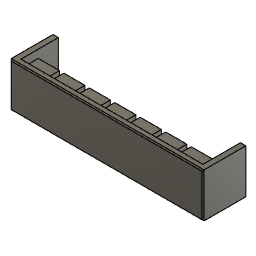
Mornsun PSU Cover (Autodesk Fusion 360 design; units mm, degrees)
Autodesk Fusion 360 part; units mm, degrees
sketch "Sketch1" plane through (0, 0, 0) normal (0, 0, 1) x (1, 0, 0) in component "Cover"
  line L0 (34, 8.25) -> (-34, 8.25)
  line L1 (-34, 8.25) -> (-34, -8.25)
  line L2 (-34, -8.25) -> (34, -8.25)
  line L3 (34, -8.25) -> (34, 8.25)
  line L4 (34, 8.25) -> (-34, -8.25) construction
  line L5 (-34, 8.25) -> (34, -8.25) construction
  line L6 (-32.5, -6.75) -> (32.5, -6.75) construction
  line L7 (32.5, -6.75) -> (32.5, 6.75) construction
  line L8 (32.5, 6.75) -> (-32.5, 6.75)
  line L9 (-32.5, 6.75) -> (-32.5, -6.75) construction
  line L10 (32.5, 4.25) -> (24.6, 4.25)
  line L11 (24.6, 4.25) -> (24.6, 6.75)
  line L12 (24.6, 6.75) -> (32.5, 6.75)
  line L13 (32.5, 6.75) -> (32.5, 4.25)
  line L14 (22.9833, 6.75) -> (22.9833, 4.25)
  line L15 (15.0833, 4.25) -> (15.0833, 6.75)
  line L16 (22.9833, 4.25) -> (15.0833, 4.25)
  line L17 (15.0833, 6.75) -> (22.9833, 6.75)
  line L18 (13.4667, 6.75) -> (13.4667, 4.25)
  line L19 (5.5667, 4.25) -> (5.5667, 6.75)
  line L20 (13.4667, 4.25) -> (5.5667, 4.25)
  line L21 (5.5667, 6.75) -> (13.4667, 6.75)
  line L22 (3.95, 6.75) -> (3.95, 4.25)
  line L23 (-3.95, 4.25) -> (-3.95, 6.75)
  line L24 (3.95, 4.25) -> (-3.95, 4.25)
  line L25 (-3.95, 6.75) -> (3.95, 6.75)
  line L26 (-5.5667, 6.75) -> (-5.5667, 4.25)
  line L27 (-13.4667, 4.25) -> (-13.4667, 6.75)
  line L28 (-5.5667, 4.25) -> (-13.4667, 4.25)
  line L29 (-13.4667, 6.75) -> (-5.5667, 6.75)
  line L30 (-15.0833, 6.75) -> (-15.0833, 4.25)
  line L31 (-22.9833, 4.25) -> (-22.9833, 6.75)
  line L32 (-15.0833, 4.25) -> (-22.9833, 4.25)
  line L33 (-22.9833, 6.75) -> (-15.0833, 6.75)
  line L34 (-24.6, 6.75) -> (-24.6, 4.25)
  line L35 (-32.5, 4.25) -> (-32.5, 6.75)
  line L36 (-24.6, 4.25) -> (-32.5, 4.25)
  line L37 (-32.5, 6.75) -> (-24.6, 6.75)
  line L38 (-34, -8.25) -> (-36, -8.25)
  line L39 (-36, -8.25) -> (-36, 8.25)
  line L40 (-36, 8.25) -> (-34, 8.25)
  line L41 (-34, 8.25) -> (-34, -8.25)
  line L42 (34, -8.25) -> (36, -8.25)
  line L43 (36, -8.25) -> (36, 8.25)
  line L44 (36, 8.25) -> (34, 8.25)
  line L45 (34, 8.25) -> (34, -8.25)
  dimension "d39" = 68
  dimension "d40" = 16.5
  dimension "d42" = 7.9
  dimension "d43" = 2.5
  dimension "d46" = -57.1
  dimension "d47" = 0
  dimension "d52" = 2
  dimension "d53" = 2
  constraint horizontal L0
  constraint perpendicular L0 L1
  constraint parallel L0 L2
  constraint parallel L1 L3
  constraint coincident L4 origin
  constraint coincident L5 origin
  constraint horizontal L10
  constraint vertical L11
  constraint horizontal L12
  constraint vertical L13
  constraint coincident L8 L11.end
  constraint coincident L7 L10.start
  constraint horizontal L38
  constraint vertical L39
  constraint horizontal L40
  constraint vertical L41
  constraint horizontal L42
  constraint vertical L43
  constraint horizontal L44
  constraint vertical L45
  measures "d39" distance of L1.end L2.end
  measures "d40" distance of L0.end L1.end
  measures "d42" distance of L10.start L10.end
  measures "d43" distance of L10.end L11.end
  measures "d52" distance of L0.start L43.end
  measures "d53" distance of L0.end L39.end
extrude "Extrude1" add sketch "Sketch1" along normal blind 2 contours L0 L1 L2 L3 L41 L45 | L3 L42 L43 L44 L45 | L1 L38 L39 L40 L41 | L8 L10 L11 L12 L13 | L8 L14 L15 L16 L17 | L8 L18 L19 L20 L21 | L8 L22 L23 L24 L25 | L8 L26 L27 L28 L29 | L8 L30 L31 L32 L33 | L8 L34 L35 L36 L37 in component "Cover"
extrude "Extrude2" add sketch "Sketch1" against normal blind 14 contours L3 L42 L43 L44 L45 | L1 L38 L39 L40 L41 in component "Cover"
extrude "Extrude3" add sketch "Sketch1" against normal blind 5 contours L8 L10 L11 L12 L13 | L8 L14 L15 L16 L17 | L8 L18 L19 L20 L21 | L8 L22 L23 L24 L25 | L8 L26 L27 L28 L29 | L8 L30 L31 L32 L33 | L8 L34 L35 L36 L37 in component "Cover"
fillet "Fillet1" radius 3 7 edges at (28.55, 4.25, 0) (19.0333, 4.25, 0) (9.5167, 4.25, 0) (0, 4.25, 0) (-9.5167, 4.25, 0) (-19.0333, 4.25, 0) (-28.55, 4.25, 0) in component "Cover"
chamfer "Chamfer1" distance 0.4 angle 45 4 edges at (-36, 0, 2) (0, 8.25, 2) (0, -8.25, 2) (36, 0, 2) in component "Cover"
component "Cover" placed x (1, 0, 0) y (0, 1, 0) z (0, 0, 1) at (0, 0, 0)
